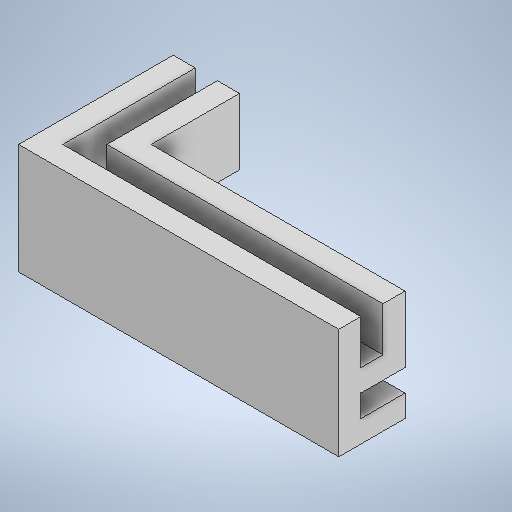
# Autodesk Inventor part: TSU_Corner1_Clamp
Saved by Autodesk Inventor 2025.2 (Build 292293000, 293)
## iProperties
Created: 2025-01-07
Part Number: TSU_Corner1_Clamp
Material: Generic
Document SubType Name: Modeling
Designer: Matt Tidd
Density: 1 g/cm^3
Appearance: Default
Author: Matt Tidd
Autodesk Inventor part; units mm, degrees
ref_plane "YZ Plane" through (0, 0, 0) normal (1, 0, 0) x (0, 1, 0)
ref_plane "XZ Plane" through (0, 0, 0) normal (0, 1, 0) x (-1, 0, 0)
ref_plane "XY Plane" through (0, 0, 0) normal (0, 0, 1) x (1, 0, 0)
sketch "Sketch1" plane through (0, 0, 0) normal (0, 1, 0) x (-1, 0, 0)
  line L0 (0, 0) -> (145, 0)
  line L1 (145, 0) -> (145, -30)
  line L2 (145, -30) -> (0, -30)
  line L3 (0, -30) -> (0, 0)
  line L4 (145, 0) -> (115, 0)
  line L5 (115, 0) -> (115, -70)
  line L6 (115, -70) -> (145, -70)
  line L7 (145, -70) -> (145, 0)
  point P0 (115, -30)
  dimension "d0" = 145
  dimension "d1" = 30
  dimension "d2" = 30
  dimension "d3" = 70
  constraints: 16 end point, 4 parallel, 2 horizontal, 2 perpendicular
  measures "d0" distance of L1.end L2.end
  measures "d1" distance of L0.end L1.end
  measures "d2" distance of L6.end L5.end
  measures "d3" distance of L5.end L4.end
extrude "Extrusion1" add sketch "Sketch1" along normal blind 30
sketch "Sketch2" plane through (0, 0, -30) normal (0, 0, -1) x (-1, 0, 0)
  line L0 (0, 20) -> (135, 20)
  line L1 (135, 20) -> (135, 10)
  line L2 (135, 10) -> (0, 10)
  line L3 (0, 10) -> (0, 20)
  dimension "d32" = 135
  dimension "d33" = 10
  constraints: 8 end point, 2 parallel, 1 horizontal, 1 perpendicular
  measures "d32" distance of L1.end L2.end
  measures "d33" distance of L0.end L1.end
extrude "Extrusion2" cut sketch "Sketch2" along normal blind 50 and the other way blind 20
sketch "Sketch4" plane through (0, 30, 0) normal (0, 1, 0) x (1, 0, 0)
  line L0 (0, 0) -> (-145, 0)
  line L1 (-145, 0) -> (-145, 10)
  line L2 (-145, 10) -> (0, 10)
  line L3 (0, 10) -> (0, 0)
  line L4 (-115, 70) -> (-145, 70) projected
  line L5 (-145, 70) -> (-135, 70)
  line L6 (-135, 70) -> (-135, 10)
  line L7 (-135, 10) -> (-145, 10)
  line L8 (-145, 10) -> (-145, 70)
  line L9 (-115, 30) -> (-115, 70) projected
  line L10 (-115, 70) -> (-125, 70)
  line L11 (-125, 70) -> (-125, 30)
  line L12 (-125, 30) -> (-115, 30)
  line L13 (-115, 30) -> (-115, 70)
  line L14 (0, 30) -> (-125, 30)
  line L15 (-125, 30) -> (-125, 20)
  line L16 (-125, 20) -> (0, 20)
  line L17 (0, 20) -> (0, 30)
  dimension "d22" = 145
  dimension "d23" = 10
  dimension "d24" = 10
  dimension "d25" = 60
  dimension "d26" = 10
  dimension "d27" = 40
  dimension "d28" = 125
  dimension "d29" = 10
  constraints: 32 end point, 8 parallel, 4 horizontal, 4 perpendicular, 2 point on line
  measures "d22" distance of L1.end L2.end
  measures "d23" distance of L0.end L1.end
  measures "d24" distance of L6.end L7.end
  measures "d25" distance of L5.end L6.end
  measures "d26" distance of L12.end L11.end
  measures "d27" distance of L11.end L10.end
  measures "d28" distance of L16.end L15.end
  measures "d29" distance of L15.end L14.end
extrude "Extrusion4" add sketch "Sketch4" along normal blind 20
body "Solid1"
